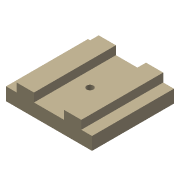
# Autodesk Inventor part: Slider
Saved by Autodesk Inventor 2015 SP1 (Build 190203100, 203)
## iProperties
Created: 2015-01-22
Part Number: Slider
Material: PET Plastic
Document SubType Name: Modeling
Designer: rihoobler
Density: 1.541 g/cm^3
Appearance: Beige
Author: rihoobler
Autodesk Inventor part; units mm, degrees
ref_plane "YZ Plane" through (0, 0, 0) normal (1, 0, 0) x (0, 1, 0)
ref_plane "XZ Plane" through (0, 0, 0) normal (0, 1, 0) x (-1, 0, 0)
ref_plane "XY Plane" through (0, 0, 0) normal (0, 0, 1) x (1, 0, 0)
sketch "Sketch1" plane through (0, 0, 0) normal (0, 0, 1) x (1, 0, 0)
  line L0 (0, 0) -> (42, 0)
  line L1 (42, 0) -> (42, 6)
  line L2 (42, 6) -> (0, 6)
  line L3 (0, 6) -> (0, 0)
  line L4 (6, 6) -> (14, 6)
  line L5 (14, 6) -> (14, 10)
  line L6 (14, 10) -> (6, 10)
  line L7 (6, 10) -> (6, 6)
  line L8 (28, 6) -> (36, 6)
  line L9 (36, 6) -> (36, 10)
  line L10 (36, 10) -> (28, 10)
  line L11 (28, 10) -> (28, 6)
  dimension "d0" = 42
  dimension "d1" = 6
  dimension "d2" = 4
  dimension "d3" = 8
  dimension "d4" = 8
  dimension "d5" = 6
  dimension "d6" = 6
  constraints: 24 end point, 6 parallel, 3 horizontal, 3 perpendicular, 3 point on line
  measures "d0" distance of L2.end L1.end
  measures "d1" distance of L0.end L1.end
  measures "d2" distance between parallel lines of L2 L6
  measures "d3" distance of L5.end L6.end
  measures "d4" distance of L9.end L10.end
  measures "d5" distance between parallel lines of L1 L9
  measures "d6" distance between parallel lines of L3 L7
extrude "Extrusion1" add sketch "Sketch1" along normal blind 38.1
sketch "Sketch2" plane through (0, 0, 0) normal (0, -1, 0) x (1, 0, 0)
  line L0 (0, 0) -> (42, 0) projected
  line L1 (0, 0) -> (0, 38.1) projected
  point P0 (21, 19.05)
  dimension "d9" = 19.05
  dimension "d10" = 21
  measures "d9" distance from line of L0 point (21, 19.05)
  measures "d10" distance from line of L1 point (21, 19.05)
hole "Hole1" at (21, 0, 19.05) direction (0, 1, 0) diameter 3.175 end through all
sketch "Sketch3" plane through (0, 0, 38.1) normal (0, 0, 1) x (1, 0, 0)
  line L0 (0, 0) -> (42, 0) projected
  line L1 (0, 6) -> (1, 6)
  line L2 (1, 6) -> (1, 0)
  line L3 (1, 0) -> (0, 0)
  line L4 (0, 0) -> (0, 6)
  line L5 (42, 6) -> (41, 6)
  line L6 (41, 6) -> (41, 0)
  line L7 (41, 0) -> (42, 0)
  line L8 (42, 0) -> (42, 6)
  dimension "d18" = 1
  dimension "d19" = 1
  constraints: 16 end point, 4 parallel, 2 horizontal, 2 perpendicular, 2 point on line
  measures "d18" distance between parallel lines of L2 L4
  measures "d19" distance between parallel lines of L8 L6
extrude "Extrusion2" cut sketch "Sketch3" against normal blind 50.8
equation "\"d4\" = d3"
equation "\"d6\" = d5"
body "Solid1"
